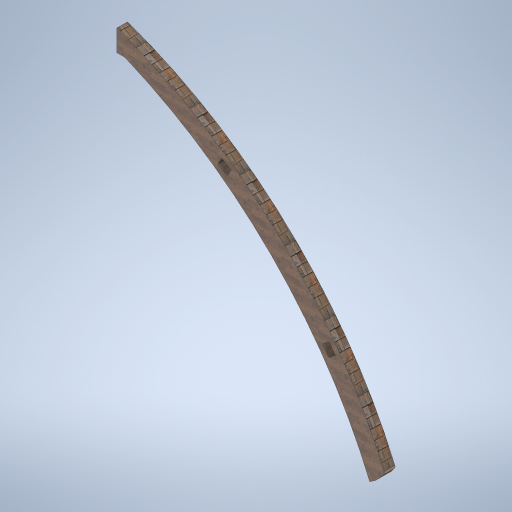
# Autodesk Inventor part: curve_beam
Saved by Autodesk Inventor 2024.2 (Build 282272000, 272)
## iProperties
Created: 2024-05-18
Part Number: curve_beam
Material: Wood Shake
Document SubType Name: Modeling
Designer: LOSTER_1
Density: 0.4 g/cm^3
Appearance: Shake - Handsplit
Author: LOSTER_1
Autodesk Inventor part; units mm, degrees
ref_plane "YZ Plane" through (0, 0, 0) normal (1, 0, 0) x (0, 1, 0)
ref_plane "XZ Plane" through (0, 0, 0) normal (0, 1, 0) x (-1, 0, 0)
ref_plane "XY Plane" through (0, 0, 0) normal (0, 0, 1) x (1, 0, 0)
sketch "Sketch2" plane through (0, 0, 0) normal (0, 0, 1) x (1, 0, 0)
  arc A0 (5000, -4000) -> (0, 700.233) centre (-2826.475, -7316.0653) ccw
  arc A1 (4600, -4000) -> (149.7898, 300.1107) centre (-3126.3122, -7543.1766) ccw
  arc A2 (4720.2587, -4274.9468) -> (4600, -4000) centre (-3126.3122, -7543.1766) ccw
  arc A3 (4720.2587, -4274.9468) -> (5000, -4000) centre (4316.4662, -3584.3299) ccw
  line L0 (149.7898, 300.1107) -> (0, 300.1107)
  line L1 (0, 300.1107) -> (0, 700.233)
  point P0 (0, 0)
  point P1 (4000, -4000)
  dimension "d5" = 8500
  dimension "d7" = 8500
  dimension "d8" = 800
  constraints: 8 point on circle, 4 centre point, 4 end point, 1 horizontal, 1 perpendicular
  measures "d5" radius of A0
  measures "d7" radius of A1
  measures "d8" radius of A3
extrude "Extrusion1" add sketch "Sketch2" along normal blind 100 and the other way blind 100
fillet "Fillet2" radius 50 2 edges at (5000, -4000, 50) (5000, -4000, -50)
sketch "Sketch4" plane through (0, 0, 100) normal (0, 0, 1) x (1, 0, 0)
  line L0 (1885.476, -557.2315) -> (2058.6811, -657.2315)
  line L1 (2058.6811, -657.2315) -> (2133.6811, -527.3277)
  line L2 (2133.6811, -527.3277) -> (1960.476, -427.3277)
  line L3 (1960.476, -427.3277) -> (1885.476, -557.2315)
  line L4 (1885.476, -557.2315) -> (2133.6811, -527.3277) construction
  line L5 (2058.6811, -657.2315) -> (1960.476, -427.3277) construction
  line L6 (1885.476, -557.2315) -> (2085.476, -557.2315) construction
  line L7 (3842.8395, -2478.8534) -> (3957.5548, -2642.6838)
  line L8 (3957.5548, -2642.6838) -> (4080.4276, -2556.6473)
  line L9 (4080.4276, -2556.6473) -> (3965.7123, -2392.8169)
  line L10 (3965.7123, -2392.8169) -> (3842.8395, -2478.8534)
  line L11 (3842.8395, -2478.8534) -> (4080.4276, -2556.6473) construction
  line L12 (3957.5548, -2642.6838) -> (3965.7123, -2392.8169) construction
  line L13 (3842.8395, -2478.8534) -> (4042.8395, -2478.8534) construction
  point P0 (0, 0)
  point P1 (2009.5785, -542.2796)
  point P2 (3961.6335, -2517.7503)
  dimension "d16" = 200
  dimension "d17" = 30
  dimension "d18" = 150
  dimension "d19" = 200
  dimension "d20" = 55
  dimension "d21" = 150
  constraints: 28 end point, 4 midpoint, 4 parallel, 2 equal length, 2 horizontal, 2 perpendicular
  measures "d16" distance of L0.start L0.end
  measures "d17" angle of L0 L6
  measures "d18" distance of L1.end L0.end
  measures "d19" distance of L7.start L7.end
  measures "d20" angle of L7 L13
  measures "d21" distance of L8.end L7.end
extrude "Extrusion2" cut sketch "Sketch4" against normal through all
body "Solid1"
